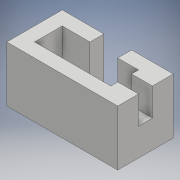
# Autodesk Inventor part: P3-3
Saved by Autodesk Inventor 2017 (Build 210142000, 142)
## iProperties
Created: 2017-02-10
Part Number: P3-3
Material: Generic
Document SubType Name: Modeling
Designer: Schaffel
Density: 1 g/cm^3
Appearance: Default
Author: Schaffel
Autodesk Inventor part; units mm, degrees
ref_plane "YZ Plane" through (0, 0, 0) normal (1, 0, 0) x (0, 1, 0)
ref_plane "XZ Plane" through (0, 0, 0) normal (0, 1, 0) x (-1, 0, 0)
ref_plane "XY Plane" through (0, 0, 0) normal (0, 0, 1) x (1, 0, 0)
sketch "Sketch1" plane through (0, 0, 0) normal (0, 0, 1) x (1, 0, 0)
  line L0 (0, 0) -> (80, 0)
  line L1 (80, 0) -> (80, 40)
  line L2 (80, 40) -> (50, 40)
  line L3 (50, 40) -> (50, 30)
  line L4 (50, 30) -> (65, 30)
  line L5 (65, 30) -> (65, 10)
  line L6 (65, 10) -> (10, 10)
  line L7 (10, 10) -> (10, 30)
  line L8 (10, 30) -> (30, 30)
  line L9 (30, 30) -> (30, 40)
  line L10 (30, 40) -> (0, 40)
  line L11 (0, 40) -> (0, 0)
  dimension "d0" = 80
  dimension "d1" = 40
  dimension "d2" = 30
  constraints: 24 end point, 10 perpendicular, 2 point on line, 1 horizontal
  measures "d0" distance of L0.start L0.end
  measures "d1" distance of L0.end L1.end
  measures "d2" distance of L1.end L2.end
extrude "Extrusion1" add sketch "Sketch1" along normal blind 20
sketch "Sketch2" plane through (0, 0, 20) normal (0, 0, 1) x (1, 0, 0)
  line L0 (30, 30) -> (30, 40) projected
  line L1 (30, 30) -> (30, 40)
  line L2 (30, 40) -> (0, 40) projected
  line L3 (30, 40) -> (0, 40)
  line L4 (0, 40) -> (0, 0) projected
  line L5 (0, 40) -> (0, 0)
  line L6 (0, 0) -> (80, 0)
  line L7 (80, 0) -> (80, 15)
  line L8 (80, 0) -> (80, 40) projected
  line L9 (80, 15) -> (65, 15)
  line L10 (65, 10) -> (10, 10) projected
  line L11 (65, 15) -> (65, 10)
  line L12 (65, 10) -> (10, 10)
  line L13 (10, 10) -> (10, 30)
  line L14 (10, 30) -> (30, 30) projected
  line L15 (10, 30) -> (30, 30)
  line L16 (80, 40) -> (50, 40) projected
  line L17 (50, 40) -> (50, 30) projected
  line L18 (50, 40) -> (50, 30)
  line L19 (50, 30) -> (65, 30) projected
  line L20 (50, 30) -> (65, 30)
  line L21 (65, 30) -> (65, 25)
  line L22 (65, 30) -> (65, 10) projected
  line L23 (65, 25) -> (80, 25)
  line L24 (80, 25) -> (80, 40)
  line L25 (50, 40) -> (80, 40)
  constraints: 32 end point, 8 collinear, 5 perpendicular, 3 point on line, 1 horizontal
extrude "Extrusion2" add sketch "Sketch2" along normal blind 20 contours L14 L13 L10 L11 L9 L7 L6 L4 L2 L0 | L21 L19 L17 L16 L8 L23
body "Solid1"
